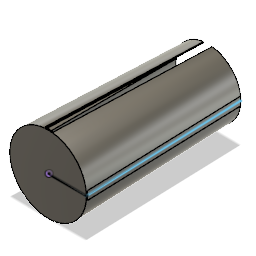
Cable Case V2 v1 (Autodesk Fusion 360 design; units mm, degrees)
Autodesk Fusion 360 part; units mm, degrees
sketch "Sketch1" plane through (0, 0, 0) normal (0, 1, 0) x (1, 0, 0)
  line L0 (0, -1) -> (0, 0)
  line L1 (0, -1) -> (35, -1)
  line L2 (35, -1) -> (36, -1)
  line L3 (30, 149) -> (31, 149)
  line L4 (31, 149) -> (36, -1)
  line L5 (35, -1) -> (30, 149)
  line L6 (0, 0) -> (35.9667, 0)
  dimension "d2" = 1
  dimension "d6" = 35
  dimension "d7" = 1
  dimension "d10" = 1
  constraint vertical L0
  constraint coincident L0.end L6.start
  constraint perpendicular L0 L1
  constraint parallel L1 L2
  constraint horizontal L3
  constraint coincident L4 L6.end
  constraint perpendicular L0 L6
  measures "d2" distance of L0.end L0.start
  measures "d6" distance of L0.start L1.end
  measures "d7" distance of L1.end L2.end
  measures "d10" distance of L3.start L3.end
revolve "Revolve1" add sketch "Sketch1" angle 360 about axis through (0, 0, 1) along (0, 0, -1)
sketch "Sketch2" plane through (0, 0, -149) normal (0, 0, -1) x (-1, 0, 0)
  circle A0 centre (0, 0) radius 30
  circle A1 centre (0, 0) radius 31
  line L0 (0, 0) -> (4, 0)
  line L1 (4, 0) -> (4, 42)
  line L2 (4, 42) -> (0, 42)
  line L3 (0, 42) -> (0, 0)
  line L4 (0, 42) -> (-4, 42)
  line L5 (-4, 42) -> (-4, 0)
  line L6 (-4, 0) -> (0, 0)
  line L7 (0, 0) -> (0, 42)
  dimension "d12" = 4
  constraint horizontal L0
  constraint vertical L1
  constraint horizontal L2
  constraint vertical L3
  constraint coincident A0.centre A1.centre
  constraint horizontal L4
  constraint vertical L5
  constraint horizontal L6
  constraint vertical L7
  measures "d12" distance of L2.end L4.end
extrude "Extrude1" cut sketch "Sketch2" against normal blind 149 contours A0 L0 L1 L3 L7 | A0 A1 L1 L3 L7 | A0 A1 L3 L5 L7 | A0 L3 L5 L6 L7 | A1 L1 L2 L3 L7 | A1 L3 L4 L5 L7
sketch "Sketch3" plane through (0, 0, -149) normal (0, 0, -1) x (-1, 0, 0)
  line L0 (4, 30.7409) -> (4, 29.7321)
  arc A0 (-4, 29.7321) -> (4, 29.7321) centre (0, 0) ccw
  line L1 (-4, 29.7321) -> (-4, 30.7409)
  arc A1 (-4, 30.7409) -> (4, 30.7409) centre (0, 0) ccw
  line L2 (0, 0) -> (-29.9997, -0.1415)
  line L3 (-28.0641, -0.1324) -> (-28.083, 3.8676)
  line L4 (-28.0641, -0.1324) -> (-28.0453, -4.1323)
  line L5 (-28.0453, -4.1323) -> (-29.7129, -4.1402)
  line L6 (-28.083, 3.8676) -> (-29.7507, 3.8597)
  line L7 (-29.7507, 3.8597) -> (-28.083, 3.8676)
  line L8 (-29.7507, 3.8597) -> (-44.7507, 3.8597)
  line L9 (-44.7507, 3.8597) -> (-44.7507, -4.1403)
  line L10 (-44.7507, -4.1403) -> (-29.7507, -4.1403)
  line L11 (-29.7507, -4.1403) -> (-29.7507, 3.8597)
  dimension "d15" = 4
  dimension "d16" = 4
  dimension "d17" = 8
  dimension "d18" = 15
  constraint coincident A0.centre A1.centre
  constraint coincident A0 L2.end
  constraint coincident L2 L3.start
  constraint perpendicular L2 L3
  constraint perpendicular L2 L4
  constraint coincident A0 L5.end
  constraint perpendicular L4 L5
  constraint coincident A0 L6.end
  constraint perpendicular L3 L6
  constraint parallel L6 L7
  constraint horizontal L8
  constraint vertical L9
  constraint horizontal L10
  constraint vertical L11
  measures "d15" distance of L3.start L3.end
  measures "d16" distance of L3.start L4.end
  measures "d17" distance of L6.end L10.end
  measures "d18" distance of L6.end L8.end
extrude "Extrude2" add sketch "Sketch3" against normal blind 149 contours A1 L8 L9 L10 | A0 A1 L8 L10 L11
sketch "Sketch4" plane through (0, 0, -149) normal (0, 0, -1) x (-1, 0, 0)
  arc A0 (-4, 29.7321) -> (-29.7507, 3.8597) centre (0, 0) ccw
  line L0 (-4, 29.7321) -> (-4, 30.7409)
  arc A1 (-4, 30.7409) -> (-30.7588, 3.8597) centre (0, 0) ccw
  line L1 (-30.7588, 3.8597) -> (-44.7507, 3.8597)
  line L2 (-44.7507, 3.8597) -> (-44.7507, -4.1403)
  line L3 (-44.7507, -4.1403) -> (-30.7223, -4.1403)
  arc A2 (-30.7223, -4.1403) -> (4, 30.7409) centre (0, 0) ccw
  line L4 (4, 30.7409) -> (4, 29.7321)
  arc A3 (-29.7507, -3.8597) -> (4, 29.7321) centre (0, 0) ccw
  arc A4 (-29.7507, 3.8597) -> (-29.7507, -3.8597) centre (0, 0) ccw
  line L5 (0, 0) -> (0, -1)
  line L6 (0, -1) -> (0, -40)
  line L7 (0, -40) -> (0, -25)
  line L8 (0, -25) -> (-4, -25)
  line L9 (-4, -25) -> (-4, -40)
  line L10 (-4, -29.7321) -> (4, -29.7321)
  line L11 (4, -29.7321) -> (4, -44.7321)
  line L12 (4, -44.7321) -> (-4, -44.7321)
  line L13 (-4, -44.7321) -> (-4, -29.7321)
  dimension "d21" = 8
  dimension "d22" = 15
  constraint coincident A0.centre A1.centre
  constraint vertical L5
  constraint parallel L5 L6
  constraint coincident L6 L7.end
  constraint parallel L6 L7
  constraint perpendicular L7 L8
  constraint perpendicular L8 L9
  constraint horizontal L10
  constraint vertical L11
  constraint horizontal L12
  constraint vertical L13
  constraint coincident L9 L10.start
  constraint coincident A3 L10.start
  measures "d21" distance of L10.start L10.end
  measures "d22" distance of L10.start L12.end
extrude "Extrude3" add sketch "Sketch4" against normal blind 149 contours A2 A3 L6 L7 L9 L13 | A2 A3 L6 L7 L11 | A2 L9 L11 L12 L13
sketch "Sketch5" plane through (0, 0, -149) normal (0, 0, -1) x (-1, 0, 0)
  arc A0 (-29.7507, -3.8597) -> (-4, -29.7321) centre (0, 0) ccw
  arc A1 (-29.7507, 3.8597) -> (-29.7507, -3.8597) centre (0, 0) ccw
  arc A2 (-4, 29.7321) -> (-29.7507, 3.8597) centre (0, 0) ccw
  line L0 (-4, 29.7321) -> (-4, 30.7409)
  arc A3 (-4, 30.7409) -> (-30.7588, 3.8597) centre (0, 0) ccw
  line L1 (-30.7588, 3.8597) -> (-44.7507, 3.8597)
  line L2 (-44.7507, 3.8597) -> (-44.7507, -4.1403)
  line L3 (-44.7507, -4.1403) -> (-30.7223, -4.1403)
  arc A4 (-30.7223, -4.1403) -> (-4, -30.7409) centre (0, 0) ccw
  line L4 (-4, -30.7409) -> (-4, -44.7321)
  line L5 (-4, -44.7321) -> (4, -44.7321)
  line L6 (4, -44.7321) -> (4, -30.7409)
  arc A5 (4, -30.7409) -> (4, 30.7409) centre (0, 0) ccw
  line L7 (4, 30.7409) -> (4, 29.7321)
  arc A6 (4, -29.7321) -> (4, 29.7321) centre (0, 0) ccw
  arc A7 (-4, -29.7321) -> (4, -29.7321) centre (0, 0) ccw
  line L8 (0, 0) -> (30, 0)
  line L9 (21.2253, 0) -> (21.2253, -4)
  line L10 (21.2253, -4) -> (41.3424, -4)
  line L11 (41.3424, -4) -> (29.7321, -4)
  line L12 (21.2253, -4) -> (41.2253, -4)
  line L13 (41.2253, -4) -> (41.2253, 4)
  line L14 (41.2253, 4) -> (21.2253, 4)
  line L15 (21.2253, 4) -> (21.2253, -4)
  dimension "d25" = 4
  dimension "d26" = 20
  dimension "d27" = 8
  constraint coincident A0.centre A1.centre
  constraint midpoint A6 L8.end
  constraint coincident L8 L9.start
  constraint perpendicular L8 L9
  constraint perpendicular L9 L10
  constraint coincident L10 L11.end
  constraint coincident A6 L11.end
  constraint horizontal L12
  constraint vertical L13
  constraint horizontal L14
  constraint vertical L15
  measures "d25" distance of L9.start L9.end
  measures "d26" distance of L9.end L12.end
  measures "d27" distance of L9.end L14.end
extrude "Extrude4" add sketch "Sketch5" against normal blind 149 contours A5 A6 L10 L11 L12 L14 | A5 L10 L11 L12 L13 L14
extrude "Extrude5" cut 3 faces at (41.8227, -0.0935, 0) (-39.4642, 0.4453, 0) (-0.4453, -41.802, 0) along direction (0, 0, -1) blind 149
extrude "Extrude6" cut 1 faces at (32.8193, 3.8597, -137.2757) along direction (0, -1, 0) blind 20
extrude "Extrude7" cut 1 faces at (-33.2112, 4, -125.1023) along direction (0, -1, 0) blind 15
extrude "Extrude8" cut 1 faces at (-4, -32.8024, -137.2764) along direction (1, 0, 0) blind 35
extrude "Extrude9" cut 1 faces at (-1.3333, -35.7435, -49.6667) along direction (0, -1, 0) blind 5
extrude "Extrude10" cut 1 faces at (-35.7435, -1.3333, -99.3333) along direction (-1, 0, 0) blind 20
extrude "Extrude11" cut 1 faces at (35.759, -1.2866, -49.6667) along direction (1, 0, 0) blind 15
equation "d40 = 3.852 mm + 0.5 mm"
equation "d42 = 3.852 mm + 0.5 mm"
equation "d44 = 5.00 mm + 0.5 mm"
